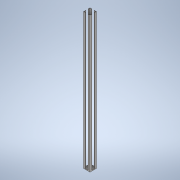
# Autodesk Inventor part: marble_lift_outer
Saved by Autodesk Inventor 2020 (Build 240168000, 168)
## iProperties
Created: 2021-03-06
Part Number: marble_lift_outer
Material: Generic
Document SubType Name: Modeling
Designer: Harry
Density: 1 g/cm^3
Appearance: Knurled 45
Author: Harry
Autodesk Inventor part; units mm, degrees
ref_plane "YZ Plane" through (0, 0, 0) normal (1, 0, 0) x (0, 1, 0)
ref_plane "XZ Plane" through (0, 0, 0) normal (0, 1, 0) x (-1, 0, 0)
ref_plane "XY Plane" through (0, 0, 0) normal (0, 0, 1) x (1, 0, 0)
sketch "Sketch1" plane through (0, 0, 0) normal (0, 1, 0) x (-1, 0, 0)
  line L0 (-19, -19) -> (19, -19)
  line L1 (19, -19) -> (19, 19)
  line L2 (19, 19) -> (-19, 19)
  line L3 (-19, 19) -> (-19, -19)
  line L4 (-19, -19) -> (19, 19) construction
  line L5 (19, -19) -> (-19, 19) construction
  point P0 (0, 0)
  dimension "d0" = 38
  dimension "d1" = 38
  constraints: 12 end point, 2 midpoint, 2 parallel, 1 horizontal, 1 perpendicular
  measures "d0" distance of L2.end L1.end
  measures "d1" distance of L1.end L0.end
extrude "Extrusion1" add sketch "Sketch1" along normal blind 5
sketch "Sketch5" plane through (0, 5, 0) normal (0, 1, 0) x (1, 0, 0)
  line L0 (-19, -19) -> (19, -19) projected
  line L1 (-19, 19) -> (19, 19)
  line L2 (19, 19) -> (19, -19)
  line L3 (19, -19) -> (-19, -19)
  line L4 (-19, -19) -> (-19, 19)
  line L5 (-19, 19) -> (19, -19) construction
  line L6 (19, 19) -> (-19, -19) construction
  point P0 (0, 0)
  constraints: 12 end point, 2 midpoint, 2 parallel, 1 horizontal, 1 perpendicular
extrude "Extrusion5" add sketch "Sketch5" along normal blind 800
sketch "Sketch6" plane through (0, 805, 0) normal (0, 1, 0) x (1, 0, 0)
  line L0 (-7.5, 27.5) -> (7.5, 27.5)
  line L1 (7.5, -27.5) -> (-7.5, -27.5)
  line L2 (-7.5, 27.5) -> (7.5, -27.5) construction
  line L3 (7.5, 27.5) -> (-7.5, -27.5) construction
  line L4 (-27.5, 7.5) -> (-27.5, -7.5)
  line L5 (27.5, -7.5) -> (27.5, 7.5)
  line L6 (27.5, 7.5) -> (-27.5, -7.5) construction
  line L7 (-27.5, 7.5) -> (27.5, -7.5) construction
  line L8 (-27.5, -7.5) -> (-7.5, -7.5)
  line L9 (7.5, -7.5) -> (27.5, -7.5)
  line L10 (7.5, 27.5) -> (7.5, 7.5)
  line L11 (7.5, -7.5) -> (7.5, -27.5)
  line L12 (27.5, 7.5) -> (7.5, 7.5)
  line L13 (-7.5, 7.5) -> (-27.5, 7.5)
  line L14 (-7.5, -27.5) -> (-7.5, -7.5)
  line L15 (-7.5, 7.5) -> (-7.5, 27.5)
  point P0 (0, 0)
  dimension "d20" = 15
  dimension "d21" = 55
  dimension "d22" = 55
  dimension "d23" = 15
  constraints: 32 end point, 10 parallel, 4 midpoint, 4 perpendicular, 3 horizontal
  measures "d20" distance of L1.start L1.end
  measures "d21" distance of L0.end L1.start
  measures "d22" distance of L5.start L4.end
  measures "d23" distance of L4.end L4.start
sketch "Sketch7" plane through (0, 805, 0) normal (0, 1, 0) x (1, 0, 0)
  line L0 (-17.5, 17.5) -> (17.5, 17.5)
  line L1 (17.5, 17.5) -> (17.5, -17.5)
  line L2 (17.5, -17.5) -> (-17.5, -17.5)
  line L3 (-17.5, -17.5) -> (-17.5, 17.5)
  line L4 (-17.5, 17.5) -> (17.5, -17.5) construction
  line L5 (17.5, 17.5) -> (-17.5, -17.5) construction
  point P0 (0, 0)
  dimension "d24" = 35
  dimension "d25" = 35
  constraints: 12 end point, 2 midpoint, 2 parallel, 1 horizontal, 1 perpendicular
  measures "d24" distance of L1.end L2.end
  measures "d25" distance of L0.end L1.end
extrude "Extrusion6" cut sketch "Sketch7" against normal blind 800
extrude "Extrusion7" cut sketch "Sketch6" against normal blind 800
sketch "Sketch8" plane through (0, 5, 0) normal (0, 1, 0) x (1, 0, 0)
  circle A0 centre (0, 0) radius 5
  dimension "d30" = 10
  constraints: 1 centre point, 1 coincident
  measures "d30" diameter of A0
extrude "Extrusion8" cut sketch "Sketch8" against normal blind 2
body "Solid1"
